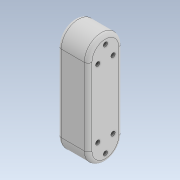
# Autodesk Inventor part: thigh
Saved by Autodesk Inventor 2020 (Build 240168000, 168)
## iProperties
Created: 2020-12-24
Part Number: thigh
Material: Generic
Document SubType Name: Modeling
Designer: DELL
Density: 1 g/cm^3
Appearance: Default
Author: DELL
Autodesk Inventor part; units mm, degrees
ref_plane "YZ Plane" through (0, 0, 0) normal (1, 0, 0) x (0, 1, 0)
ref_plane "XZ Plane" through (0, 0, 0) normal (0, 1, 0) x (-1, 0, 0)
ref_plane "XY Plane" through (0, 0, 0) normal (0, 0, 1) x (1, 0, 0)
sketch "Sketch1" plane through (0, 0, 0) normal (1, 0, 0) x (0, 1, 0)
  arc A0 (0, -22.5) -> (0, 22.5) centre (0, 0) ccw
  arc A1 (-100, 22.5) -> (-100, -22.5) centre (-100, 0) ccw
  line L0 (0, 22.5) -> (-100, 22.5)
  line L1 (0, -22.5) -> (-100, -22.5)
  circle A2 centre (0, 0) radius 11.5 construction
  line L2 (22.5, 0) -> (0, 0) construction
  line L3 (0, 0) -> (-7.125, 12.3409) construction
  line L4 (0, 0) -> (-7.125, -12.3409) construction
  line L5 (0, 22.5) -> (0, -22.5) construction
  circle A3 centre (11.5, 0) radius 1.65
  circle A4 centre (-5.75, 9.9593) radius 1.65
  circle A5 centre (-5.75, -9.9593) radius 1.65
  circle A6 centre (11.5, 0) radius 2.75
  circle A7 centre (-5.75, -9.9593) radius 2.75
  circle A8 centre (-5.75, 9.9593) radius 2.75
  line L6 (0, 0) -> (5.8575, 10.1455) construction
  line L7 (0, 0) -> (5.8575, -10.1455) construction
  circle A9 centre (0, 0) radius 9.715 construction
  circle A10 centre (4.8575, 8.4134) radius 2
  circle A11 centre (4.8575, -8.4134) radius 2
  circle A12 centre (-9.715, 0) radius 2
  line L8 (-50, 22.5) -> (-50, -22.5) construction
  circle A13 centre (-111.5, 0) radius 1.65
  circle A14 centre (-94.25, 9.9593) radius 1.65
  circle A15 centre (-94.25, -9.9593) radius 1.65
  circle A16 centre (-111.5, 0) radius 2.75
  circle A17 centre (-94.25, -9.9593) radius 2.75
  circle A18 centre (-94.25, 9.9593) radius 2.75
  circle A19 centre (-104.8575, 8.4134) radius 2
  circle A20 centre (-104.8575, -8.4134) radius 2
  circle A21 centre (-90.285, 0) radius 2
  line L9 (-50, -22.5) -> (-50, 22.5)
  point P0 (0, 0)
  dimension "d6" = 4
  dimension "d0" = 23
  dimension "d1" = 30
  dimension "d2" = 3.3
  dimension "d3" = 5.5
  dimension "d4" = 30
  dimension "d5" = 19.43
  dimension "d7" = 45
  dimension "d8" = 100
  constraints: 20 end point, 18 centre point, 11 point on circle, 9 coincident, 9 symmetric about line, 5 point on line, 4 tangent, 3 equal radius, 3 midpoint, 2 horizontal alignment, 1 collinear, 1 horizontal, 1 vertical, 25 other
  measures "d0" diameter of A2
  measures "d1" angle of L3 L5
  measures "d2" diameter of A3
  measures "d3" diameter of A6
  measures "d4" angle of L5 L6
  measures "d5" diameter of A9
  measures "d7" diameter of A0
  measures "d8" distance of A1.centre point (0, 0)
extrude "Extrusion1" add sketch "Sketch1" along normal mid plane 40 contours L1 L9 L0 A0 | A6 | A7 | A8 | A10 | A11 | A12
extrude "Extrusion2" cut sketch "Sketch1" against normal blind 35 from surface at 20 contours A6 | A7 | A8
extrude "Extrusion3" cut sketch "Sketch1" along normal blind 5 from surface at -20 contours A10 | A11 | A12
ref_plane "Work Plane1" through (0, -50, 22.5) normal (0, -1, 0) x (0, 0, -1)
mirror "Mirror1" about plane through (0, -50, 22.5) normal (0, -1, 0)
fillet "Fillet1" radius 5 8 edges at (-20, -122.5, 0) (-20, -50, -22.5) (-20, 22.5, 0) (-20, -50, 22.5) (20, -122.5, 0) (20, -50, -22.5) (20, 22.5, 0) (20, -50, 22.5)
body "Solid1"
